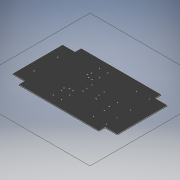
# Autodesk Inventor part: 000.001.002 - Днище
Saved by Autodesk Inventor 2022 (Build 260153000, 153)
## iProperties
Created: 2022-02-23
Part Number: 000.001.002 - Днище
Material: Типовые
Document SubType Name: Modeling
Designer: Petrov Ivan
Density: 1 g/cm^3
Appearance: По умолчанию(1)
Author: Petrov Ivan
Autodesk Inventor part; units mm, degrees
ref_plane "YZ Plane" through (0, 0, 0) normal (1, 0, 0) x (0, 1, 0)
ref_plane "XZ Plane" through (0, 0, 0) normal (0, 1, 0) x (-1, 0, 0)
ref_plane "XY Plane" through (0, 0, 0) normal (0, 0, 1) x (1, 0, 0)
sketch "Эскиз1" plane through (0, 0, 0) normal (0, 1, 0) x (-1, 0, 0)
  line L0 (-238, 142) -> (238, 142)
  line L1 (238, 142) -> (238, -142)
  line L2 (238, -142) -> (-238, -142)
  line L3 (-238, -142) -> (-238, 142)
  line L4 (-238, 142) -> (238, -142) construction
  line L5 (238, 142) -> (-238, -142) construction
  circle A0 centre (-139.231, 22.646) radius 2
  point P0 (0, 0)
  dimension "d0" = 476
  dimension "d1" = 284
  dimension "d10" = 4
  constraints: 12 end point, 2 midpoint, 2 parallel, 1 centre point, 1 horizontal, 1 perpendicular
  measures "d0" distance of L1.end L2.end
  measures "d1" distance of L0.end L1.end
  measures "d10" diameter of A0
extrude "Выдавливание1" add sketch "Эскиз1" along normal blind 4 contours L0 L1 L2 L3 | A0
sketch "Эскиз2" plane through (0, 4, 0) normal (0, 1, 0) x (1, 0, 0)
  line L0 (-238, -142) -> (238, -142) projected
  line L1 (-238, -142) -> (-182, -142)
  line L2 (-182, -142) -> (-182, -114)
  line L3 (-182, -114) -> (-238, -114)
  line L4 (-238, -114) -> (-238, -142)
  point P0 (0, 0)
  dimension "d4" = 56
  dimension "d5" = 28
  constraints: 8 end point, 2 parallel, 1 horizontal, 1 perpendicular
  measures "d4" distance of L3.end L2.end
  measures "d5" distance of L2.end L1.end
extrude "Выдавливание2" cut sketch "Эскиз2" against normal blind 4
mirror "Зеркальное отражение1" about plane through (0, 0, 0) normal (1, 0, 0) of "Выдавливание2"
mirror "Зеркальное отражение2" about plane through (0, 0, 0) normal (0, 0, 1) of "Выдавливание2", "Зеркальное отражение1"
sketch "Эскиз3" plane through (0, 0, 0) normal (0, -1, 0) x (1, 0, 0)
  circle A0 centre (114, -97) radius 1.375 projected
  circle A1 centre (172, -97) radius 1.375 projected
  circle A2 centre (172, -11) radius 1.375 projected
  circle A3 centre (114, -11) radius 1.375 projected
  circle A4 centre (172.5, 49.5) radius 1.35 projected
  circle A5 centre (172.5, 98.5) radius 1.35 projected
  circle A6 centre (114.5, 98.5) radius 1.35 projected
  circle A7 centre (114.5, 49.5) radius 1.35 projected
  point P0 (0, 0)
extrude "Выдавливание3" cut sketch "Эскиз3" against normal through all
sketch "Эскиз4" plane through (0, 0, 0) normal (0, -1, 0) x (1, 0, 0)
  circle A0 centre (110.1908, 22.1766) radius 2
  point P0 (0, 0)
  dimension "d11" = 4
  constraints: 1 centre point
  measures "d11" diameter of A0
extrude "Выдавливание4" cut sketch "Эскиз4" against normal blind 10
pattern_linear "Прямоуг.массив1" count 3 spacing 60 along (-1, 0, 0) of "Выдавливание4"
sketch "Эскиз5" plane through (0, 0, 0) normal (0, -1, 0) x (1, 0, 0)
  circle A0 centre (-34.2279, 43.4021) radius 2
  circle A1 centre (-49.5827, 43.4021) radius 2
  point P0 (0, 0)
  dimension "d17" = 4
  dimension "d18" = 4
  constraints: 2 centre point, 1 horizontal alignment
  measures "d17" diameter of A0
  measures "d18" diameter of A1
extrude "Выдавливание5" cut sketch "Эскиз5" against normal blind 10
mirror "Зеркальное отражение3" about plane through (0, 0, 0) normal (0, 0, 1) of "Выдавливание5"
sketch "Эскиз6" plane through (0, 0, 0) normal (0, -1, 0) x (1, 0, 0)
  circle A0 centre (-24.25, 67.625) radius 1.5 projected
  circle A1 centre (-24.25, 104.625) radius 1.5 projected
  circle A2 centre (-61.25, 104.625) radius 1.5 projected
  circle A3 centre (-61.25, 67.625) radius 1.5 projected
  circle A4 centre (-61.25, -67.625) radius 1.5 projected
  circle A5 centre (-24.25, -67.625) radius 1.5 projected
  circle A6 centre (-24.25, -104.625) radius 1.5 projected
  circle A7 centre (-61.25, -104.625) radius 1.5 projected
  point P0 (0, 0)
extrude "Выдавливание6" cut sketch "Эскиз6" against normal blind 10
sketch "Эскиз7" plane through (0, 0, 0) normal (0, -1, 0) x (1, 0, 0)
  circle A0 centre (-64.5827, -53.4021) radius 2 projected
  circle A1 centre (-64.5827, 53.4019) radius 2 projected
  circle A2 centre (-199.5827, -53.4021) radius 2 projected
  circle A3 centre (-199.5827, 53.4019) radius 2 projected
  point P0 (0, 0)
extrude "Выдавливание7" cut sketch "Эскиз7" against normal blind 10
sketch "Эскиз8" plane through (0, 0, 0) normal (0, -1, 0) x (1, 0, 0)
  circle A0 centre (-12.2692, -21.9834) radius 1.5 projected
  circle A1 centre (-12.2692, 2.1466) radius 1.5 projected
  circle A2 centre (42.3408, 2.1466) radius 1.5 projected
  circle A3 centre (42.3408, -21.9834) radius 1.5 projected
  point P0 (0, 0)
extrude "Выдавливание8" cut sketch "Эскиз8" against normal blind 10
